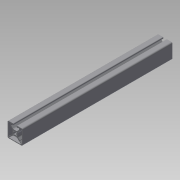
# Autodesk Inventor part: 1501-LS
Saved by Autodesk Inventor 2013 (Build 170138000, 138)
## iProperties
Created: 2014-04-23
Part Number: 1501-LS
Material: Generic
Document SubType Name: Modeling
Density: 1 g/cm^3
Vendor: 80/20 Inc.
Engineer: Ross Bowman
Designer: Ross Bowman
Catalog Web Link: 8020.net
Company: 80/20 Inc.
Author: Ross Bowman
Keywords: 80/20 , 8020 , T-Slot , Extrusion
Material: 6105-T5 Aluminum
Autodesk Inventor part; units mm, degrees
ref_plane "YZ Plane" through (0, 0, 0) normal (1, 0, 0) x (0, 1, 0)
ref_plane "XZ Plane" through (0, 0, 0) normal (0, 1, 0) x (-1, 0, 0)
ref_plane "XY Plane" through (0, 0, 0) normal (0, 0, 1) x (1, 0, 0)
sketch "Sketch1" plane through (0, 0, 0) normal (0, 0, 1) x (1, 0, 0)
  arc A0 (-4.3433, -2.7269) -> (-2.7269, -4.3433) centre (-3.5351, -3.5351) ccw
  line L0 (-2.9729, -1.3564) -> (-4.3433, -2.7269)
  arc A1 (-2.9729, 1.3564) -> (-2.9729, -1.3564) centre (0, 0) ccw
  line L1 (-4.3433, 2.7269) -> (-2.9729, 1.3564)
  arc A2 (-2.7269, 4.3433) -> (-4.3433, 2.7269) centre (-3.5351, 3.5351) ccw
  line L2 (-1.3564, 2.9729) -> (-2.7269, 4.3433)
  arc A3 (1.3564, 2.9729) -> (-1.3564, 2.9729) centre (0, 0) ccw
  line L3 (2.6398, 4.2456) -> (1.3564, 2.9729)
  arc A4 (4.2456, 2.6398) -> (2.6398, 4.2456) centre (3.5351, 3.5351) ccw
  line L4 (2.9729, 1.3564) -> (4.2456, 2.6398)
  arc A5 (2.9729, -1.3564) -> (2.9729, 1.3564) centre (0, 0) ccw
  line L5 (4.3433, -2.7269) -> (2.9729, -1.3564)
  arc A6 (2.7269, -4.3433) -> (4.3433, -2.7269) centre (3.5351, -3.5351) ccw
  line L6 (1.3564, -2.9729) -> (2.7269, -4.3433)
  arc A7 (-1.3564, -2.9729) -> (1.3564, -2.9729) centre (0, 0) ccw
  line L7 (-2.7269, -4.3433) -> (-1.3564, -2.9729)
  arc A8 (16.5959, -15.3395) -> (17.2463, -15.0701) centre (16.8653, -15.0701) ccw
  line L8 (12.2199, -10.963) -> (16.5959, -15.3395)
  arc A9 (11.9967, -10.4242) -> (12.2199, -10.963) centre (12.7587, -10.4242) ccw
  line L9 (11.9967, -10.1574) -> (11.9967, -10.4242)
  arc A10 (11.9967, -10.1574) -> (11.7735, -9.6186) centre (11.2347, -10.1574) ccw
  line L10 (8.2569, -6.1016) -> (11.7735, -9.6186)
  arc A11 (6.8659, -2.7433) -> (8.2569, -6.1016) centre (11.6157, -2.7432) ccw
  line L11 (6.8657, 2.742) -> (6.8659, -2.7433)
  arc A12 (8.2571, 6.1009) -> (6.8657, 2.742) centre (11.6155, 2.7421) ccw
  line L12 (11.2694, 9.1129) -> (8.2571, 6.1009)
  arc A13 (11.2694, 9.1129) -> (12.1994, 11.3582) centre (9.0244, 11.3581) ccw
  line L13 (12.1992, 16.8653) -> (12.1994, 11.3582)
  arc A14 (12.5802, 17.2463) -> (12.1992, 16.8653) centre (12.5802, 16.8653) ccw
  line L14 (14.4539, 17.2462) -> (12.5802, 17.2463)
  arc A15 (17.2478, 14.452) -> (14.4539, 17.2462) centre (14.4538, 14.4522) ccw
  line L15 (17.2463, -15.0701) -> (17.2478, 14.452)
  arc A16 (-17.2463, -15.0701) -> (-16.5959, -15.3395) centre (-16.8653, -15.0701) ccw
  line L16 (-17.2478, 14.452) -> (-17.2463, -15.0701)
  arc A17 (-14.4539, 17.2462) -> (-17.2478, 14.452) centre (-14.4538, 14.4522) ccw
  line L17 (-12.5802, 17.2463) -> (-14.4539, 17.2462)
  arc A18 (-12.1992, 16.8653) -> (-12.5802, 17.2463) centre (-12.5802, 16.8653) ccw
  line L18 (-12.1994, 11.3582) -> (-12.1992, 16.8653)
  arc A19 (-12.1994, 11.3582) -> (-11.2694, 9.1129) centre (-9.0244, 11.3581) ccw
  line L19 (-8.2571, 6.1009) -> (-11.2694, 9.1129)
  arc A20 (-6.8657, 2.742) -> (-8.2571, 6.1009) centre (-11.6155, 2.7421) ccw
  line L20 (-6.8659, -2.7433) -> (-6.8657, 2.742)
  arc A21 (-8.2569, -6.1016) -> (-6.8659, -2.7433) centre (-11.6157, -2.7432) ccw
  line L21 (-11.7735, -9.6186) -> (-8.2569, -6.1016)
  arc A22 (-11.7735, -9.6186) -> (-11.9967, -10.1574) centre (-11.2347, -10.1574) ccw
  line L22 (-11.9967, -10.4242) -> (-11.9967, -10.1574)
  arc A23 (-12.2199, -10.963) -> (-11.9967, -10.4242) centre (-12.7587, -10.4242) ccw
  line L23 (-16.5959, -15.3395) -> (-12.2199, -10.963)
  arc A24 (-2.7432, -6.8653) -> (-6.1022, -8.2567) centre (-2.7433, -11.6151) ccw
  line L24 (2.7429, -6.8654) -> (-2.7432, -6.8653)
  arc A25 (6.1015, -8.2568) -> (2.7429, -6.8654) centre (2.7428, -11.6152) ccw
  line L25 (9.6176, -11.7732) -> (6.1015, -8.2568)
  arc A26 (9.6176, -11.7732) -> (10.1564, -11.9964) centre (10.1565, -11.2344) ccw
  line L26 (10.4232, -11.9964) -> (10.1564, -11.9964)
  arc A27 (10.962, -12.2196) -> (10.4232, -11.9964) centre (10.4231, -12.7584) ccw
  line L27 (15.3386, -16.5967) -> (10.962, -12.2196)
  arc A28 (15.0692, -17.2471) -> (15.3386, -16.5967) centre (15.0692, -16.8661) ccw
  line L28 (-15.0701, -17.2463) -> (15.0692, -17.2471)
  arc A29 (-15.3395, -16.5959) -> (-15.0701, -17.2463) centre (-15.0701, -16.8653) ccw
  line L29 (-10.963, -12.2199) -> (-15.3395, -16.5959)
  arc A30 (-10.4242, -11.9967) -> (-10.963, -12.2199) centre (-10.4242, -12.7587) ccw
  line L30 (-10.1574, -11.9967) -> (-10.4242, -11.9967)
  arc A31 (-10.1574, -11.9967) -> (-9.6185, -11.7735) centre (-10.1574, -11.2347) ccw
  line L31 (-6.1022, -8.2567) -> (-9.6185, -11.7735)
  arc A32 (6.477, 14.986) -> (6.858, 15.367) centre (6.477, 15.367) ccw
  line L32 (6.858, 15.367) -> (6.858, 15.4432)
  arc A33 (7.239, 15.8242) -> (6.858, 15.4432) centre (7.239, 15.4432) ccw
  line L33 (7.239, 15.8242) -> (9.017, 15.8242)
  arc A34 (10.287, 14.5542) -> (9.017, 15.8242) centre (9.017, 14.5542) ccw
  line L34 (10.287, 14.5542) -> (10.287, 12.9683)
  arc A35 (9.915, 12.0703) -> (10.287, 12.9683) centre (9.017, 12.9683) ccw
  line L35 (9.915, 12.0703) -> (5.9669, 8.1222)
  arc A36 (2.6083, 6.731) -> (5.9669, 8.1222) centre (2.6083, 11.4808) ccw
  line L36 (2.6083, 6.731) -> (-2.6083, 6.731)
  arc A37 (-5.9669, 8.1222) -> (-2.6083, 6.731) centre (-2.6083, 11.4808) ccw
  line L37 (-5.9669, 8.1222) -> (-9.915, 12.0703)
  arc A38 (-10.287, 12.9683) -> (-9.915, 12.0703) centre (-9.017, 12.9683) ccw
  line L38 (-10.287, 12.9683) -> (-10.287, 14.5542)
  arc A39 (-9.017, 15.8242) -> (-10.287, 14.5542) centre (-9.017, 14.5542) ccw
  line L39 (-9.017, 15.8242) -> (-7.239, 15.8242)
  arc A40 (-6.858, 15.4432) -> (-7.239, 15.8242) centre (-7.239, 15.4432) ccw
  line L40 (-6.858, 15.4432) -> (-6.858, 15.367)
  arc A41 (-6.858, 15.367) -> (-6.477, 14.986) centre (-6.477, 15.367) ccw
  line L41 (-6.477, 14.986) -> (-5.6388, 14.986)
  arc A42 (-5.6388, 14.986) -> (-4.064, 16.5608) centre (-5.6388, 16.5608) ccw
  line L42 (-4.064, 16.5608) -> (-4.064, 17.4752)
  arc A43 (-4.064, 17.4752) -> (-5.6388, 19.05) centre (-5.6388, 17.4752) ccw
  line L43 (-5.6388, 19.05) -> (-15.875, 19.05)
  arc A44 (-15.875, 19.05) -> (-19.05, 15.875) centre (-15.875, 15.875) ccw
  line L44 (-19.05, 15.875) -> (-19.05, -15.875)
  arc A45 (-19.05, -15.875) -> (-15.875, -19.05) centre (-15.875, -15.875) ccw
  line L45 (-15.875, -19.05) -> (15.875, -19.05)
  arc A46 (15.875, -19.05) -> (19.05, -15.875) centre (15.875, -15.875) ccw
  line L46 (19.05, -15.875) -> (19.05, 15.875)
  arc A47 (19.05, 15.875) -> (15.875, 19.05) centre (15.875, 15.875) ccw
  line L47 (15.875, 19.05) -> (5.6388, 19.05)
  arc A48 (5.6388, 19.05) -> (4.064, 17.4752) centre (5.6388, 17.4752) ccw
  line L48 (4.064, 17.4752) -> (4.064, 16.5608)
  arc A49 (4.064, 16.5608) -> (5.6388, 14.986) centre (5.6388, 16.5608) ccw
  line L49 (5.6388, 14.986) -> (6.477, 14.986)
  constraints: 100 end point, 100 point on circle, 50 centre point
extrude "Extrusion1" add sketch "Sketch1" against normal blind 381
body "Solid1"
